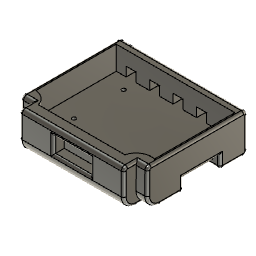
Carcasa Muñeca v10.0 (Autodesk Fusion 360 design; units mm, degrees)
Autodesk Fusion 360 part; units mm, degrees
sketch "Sketch10" plane through (0, 0, 0) normal (0, 0, 1) x (1, 0, 0)
  line L0 (0, -50) -> (0, 50) construction
  line L1 (0, 50) -> (-57, 50)
  line L2 (-57, 50) -> (-57, 0)
  line L3 (0, -50) -> (-45, -50)
  line L4 (-45, -50) -> (-45, -30)
  arc A0 (-57, 0) -> (-45, -30) centre (-7.0663, 2.5735) ccw
  line L5 (0, -50) -> (45, -50)
  line L6 (45, -50) -> (45, -30)
  arc A1 (45, -30) -> (57, 0) centre (7.0663, 2.5735) ccw
  line L7 (57, 50) -> (57, 0)
  line L8 (0, 50) -> (57, 50)
  dimension "d19" = 100
  dimension "d20" = 57
  dimension "d21" = 50
  dimension "d22" = 45
  dimension "d23" = 20
  dimension "d24" = 50
  dimension "d25" = 30
  constraint vertical L0
  constraint midpoint L0 origin
  constraint perpendicular L0 L1
  constraint perpendicular L1 L2
  constraint perpendicular L0 L3
  constraint perpendicular L3 L4
  constraint symmetric L3.start L0 L5.start
  constraint symmetric L1.start L0 L8.start
  constraint symmetric L0 L1.end L7.start
  constraint symmetric L0 L2.end A1.end
  constraint symmetric L0 L3.end L5.end
  constraint symmetric L0 L4.end L6.end
  constraint symmetric L0 A0 A1
  measures "d19" distance of L0.start L0.end
  measures "d20" distance of L0.end L1.end
  measures "d21" distance of L1.end L2.end
  measures "d22" distance of L0.start L3.end
  measures "d23" distance of L3.end L4.end
  measures "d24" radius of A0
  measures "d25" vertical distance of L2.end L4.end
sketch "Sketch12" plane through (0, 0, 0) normal (1, 0, 0) x (0, 1, 0)
  line L0 (0, 15.5) -> (0, -15.5) construction
  line L1 (0, 15.5) -> (40, 15.5)
  line L2 (43, 12.5) -> (43, -12.5)
  arc A0 (43, 12.5) -> (40, 15.5) centre (40, 12.5) ccw
  line L3 (0, 15.5) -> (-45, 15.5)
  line L4 (-48, 12.5) -> (-48, -5.5)
  arc A1 (-45, 15.5) -> (-48, 12.5) centre (-45, 12.5) ccw
  arc A2 (-48, -5.5) -> (-38, -15.5) centre (-38, -5.5) ccw
  arc A3 (40, -15.5) -> (43, -12.5) centre (40, -12.5) ccw
  line L5 (-38, -15.5) -> (40, -15.5)
  dimension "d30" = 3
  dimension "d34" = 3
  dimension "d35" = 10
  dimension "d36" = 18
  dimension "d38" = 3
  dimension "d40" = 25
  dimension "d308" = 45
  dimension "d309" = 40
  constraint vertical L0
  constraint midpoint L0 origin
  constraint perpendicular L0 L1
  constraint perpendicular L1 L2
  constraint tangent L1 A0
  constraint tangent L2 A0
  constraint perpendicular L0 L3
  constraint perpendicular L3 L4
  constraint tangent L4 A1
  constraint tangent L3 A1
  constraint tangent L4 A2
  constraint tangent L2 A3
  constraint tangent A3 L5
  measures "d30" radius of A0
  measures "d34" radius of A1
  measures "d35" radius of A2
  measures "d36" distance of L4.start L4.end
  measures "d38" radius of A3
  measures "d40" distance of L2.start L2.end
  measures "d308" distance of L0.start L3.end
  measures "d309" distance of L0.start L1.end
extrude "Extrude1" add sketch "Sketch12" along normal mid plane 84
ref_plane "PlanoDeObra18" through (-51, -2.5, 0) normal (-1, 0, 0) x (0, -1, 0)
sketch "Boceto31" plane through (-42, 0, 0) normal (-1, 0, 0) x (0, -1, 0)
  line L0 (45, 15.5) -> (-40, 15.5)
  line L1 (-43, 12.5) -> (-43, -12.5)
  arc A0 (-43, -12.5) -> (-40, -15.5) centre (-40, -12.5) ccw
  arc A1 (38, -15.5) -> (48, -5.5) centre (38, -5.5) ccw
  line L2 (48, -5.5) -> (48, 12.5)
  arc A2 (48, 12.5) -> (45, 15.5) centre (45, 12.5) ccw
  arc A3 (-43, -12.5) -> (-40, -15.5) centre (-40, -12.5) ccw
  line L3 (-40, -12.5) -> (-43, -12.5) construction
  line L4 (-40, -12.5) -> (-40, -15.5) construction
  line L5 (-40, -15.5) -> (28, -15.5)
  line L6 (-40, 15.5) -> (35, 15.5)
  line L7 (-43, 12.5) -> (-43, -12.5)
  arc A4 (38, 12.5) -> (34.9876, 15.5) centre (35, 12.5) ccw
  line L8 (35, 12.5) -> (38, 12.5) construction
  line L9 (35, 12.5) -> (34.9876, 15.5) construction
  arc A5 (28, -15.5) -> (38, -5.5) centre (28, -5.5) ccw
  line L10 (28, -5.5) -> (28, -15.5) construction
  line L11 (28, -5.5) -> (38, -5.5) construction
  line L12 (38, -5.5) -> (38, 12.5)
  line L13 (-40, -15.5) -> (38, -15.5)
  arc A6 (-40, 15.5) -> (-43, 12.4998) centre (-40, 12.5) ccw
  line L14 (-40, 12.5) -> (-40, 15.5) construction
  line L15 (-40, 12.5) -> (-43, 12.4998) construction
  dimension "d172" = 3
  dimension "d176" = 3
  dimension "d178" = 10
  dimension "d313" = 68
  dimension "d315" = 75
  dimension "d316" = 3
  dimension "d396" = 10
  constraint coincident A0.centre A3.centre
  constraint coincident A0.end A3.end
  constraint perpendicular L4 L5
  constraint parallel L0 L6
  constraint tangent A3 L7
  constraint tangent L6 A4
  constraint tangent L5 A5
  constraint tangent A5 L12
  constraint tangent A4 L12
  constraint perpendicular L6 L12
  constraint coincident L0.end L6.start
  constraint tangent L6 A6
  constraint tangent L7 A6
  measures "d172" radius of A3
  measures "d176" radius of A4
  measures "d178" radius of A5
  measures "d313" distance of A0.end L5.end
  measures "d315" distance of L0.end L6.end
  measures "d316" radius of A6
  measures "d396" distance of L2 L12
extrude "Extruir14" add sketch "Boceto31" along normal blind 9 contours L0 L1 A0 A3 L5 L6 L7 A4 A5 L12 L13 A6
sketch "Boceto32" plane through (42, 0, 0) normal (1, 0, 0) x (0, 1, 0)
  line L0 (40, 15.5) -> (-45, 15.5)
  arc A0 (-45, 15.5) -> (-48, 12.5) centre (-45, 12.5) ccw
  line L1 (-48, 12.5) -> (-48, -5.5)
  arc A1 (-48, -5.5) -> (-38, -15.5) centre (-38, -5.5) ccw
  arc A2 (40, -15.5) -> (43, -12.5) centre (40, -12.5) ccw
  line L2 (43, -12.5) -> (43, 12.5)
  arc A3 (43, 12.5) -> (40, 15.5) centre (40, 12.5) ccw
  arc A4 (43, 12.5) -> (40, 15.5) centre (40, 12.5) ccw
  line L3 (40, 12.5) -> (43, 12.5) construction
  line L4 (40, 12.5) -> (40, 15.5) construction
  line L5 (40, 15.5) -> (-35, 15.5)
  arc A5 (40, -15.5) -> (43, -12.5) centre (40, -12.5) ccw
  line L6 (40, -12.5) -> (40, -15.5) construction
  line L7 (40, -12.5) -> (43, -12.5) construction
  line L8 (-28, -15.5) -> (-28, -5.5) construction
  arc A6 (-37.9995, -5.4037) -> (-28, -15.5) centre (-28, -5.5) ccw
  line L9 (-28, -5.5) -> (-37.9995, -5.4037) construction
  line L10 (-28, -5.5) -> (-28, -15.5) construction
  arc A7 (-34.8271, 15.5) -> (-37.8271, 12.5004) centre (-34.8271, 12.5) ccw
  line L11 (-34.8271, 12.5) -> (-34.8271, 15.5) construction
  line L12 (-34.8271, 12.5) -> (-37.8271, 12.5004) construction
  line L13 (-37.8271, 12.5004) -> (-37.9995, -5.4037)
  line L14 (-28, -15.5) -> (40, -15.5)
  line L15 (-28, -15.5) -> (40, -15.5)
  line L16 (43, 12.5) -> (43, -12.5)
  dimension "d182" = 3
  dimension "d185" = 3
  dimension "d320" = 10
  dimension "d322" = 3
  dimension "d397" = 75
  dimension "d398" = 68
  constraint coincident A3.centre A4.centre
  constraint coincident L0.start A3.end
  constraint coincident A2.centre A5.centre
  constraint coincident A2.start A5.start
  constraint coincident L8.start A6.end
  constraint coincident L8.end A6.centre
  constraint tangent A6 L13
  constraint tangent L5 A7
  constraint tangent A6 L14
  measures "d182" radius of A4
  measures "d185" radius of A5
  measures "d320" radius of A6
  measures "d322" radius of A7
  measures "d397" distance of L0.start L5.end
  measures "d398" distance of A2.start L8.start
extrude "Extruir15" add sketch "Boceto32" along normal blind 9
ref_plane "PlanoDeObra19" through (0, -2.5, -0.5) normal (0, 0, 1) x (0, -1, 0)
sketch "Boceto33" plane through (0, 0, -0.5) normal (0, 0, 1) x (1, 0, 0)
  line L0 (48, 36) -> (-48, 36)
  line L1 (-48, 36) -> (-48, -29)
  line L2 (48, -29) -> (48, 36)
  line L3 (-37, -37.9882) -> (33, -37.9882)
  line L4 (-51, 40) -> (-51, -28)
  line L5 (-42, 40) -> (51, 40)
  line L6 (-42, -45) -> (42, -45)
  line L7 (-42, -45) -> (-42, -35)
  line L8 (51, 40) -> (51, -34.8271)
  arc A0 (-37, -37.9882) -> (-48, -29) centre (-48.8903, -41.3147) ccw
  arc A1 (48, -29) -> (33, -37.9882) centre (44.9809, -40.972) ccw
  line L9 (42, -34.8271) -> (42, -45)
  dimension "d257" = 3
  dimension "d310" = 4
  dimension "d325" = 70
  dimension "d327" = 65
  dimension "d330" = 3
  dimension "d399" = 5
  dimension "d400" = 9
  constraint horizontal L0
  constraint vertical L1
  constraint vertical L2
  constraint horizontal L3
  constraint equal L1 L2
  constraint equal A0 A1
  measures "d257" distance of L1 L4
  measures "d310" distance of L0 L5
  measures "d325" distance of L3.start L3.end
  measures "d327" distance of L0.end L1.end
  measures "d330" distance of L2 L8
  measures "d399" distance of L3.start L7
  measures "d400" distance of L3.end L9
extrude "Extruir16" cut sketch "Boceto33" along normal blind 16 and the other way blind 3
ref_plane "PlanoDeObra20" through (51, 2.5864, 15.5) normal (-1, 0, 0) x (0, -1, 0)
sketch "Boceto34" plane through (51, 10, 10) normal (-1, 0, 0) x (0, 0, -1)
  line L0 (25.5, 19) -> (15.5, 19)
  line L1 (15.5, 19) -> (15.5, -11)
  line L2 (15.5, -11) -> (25.5, -11)
  line L3 (25.5, -11) -> (25.5, 19)
  line L4 (25.5, 38) -> (25.5, -30)
  dimension "d205" = 10
  dimension "d206" = 30
  dimension "d331" = 19
  constraint horizontal L0
  constraint vertical L1
  constraint horizontal L2
  constraint vertical L3
  constraint coincident L2.end L4
  measures "d205" distance of L0.start L0.end
  measures "d206" distance of L0.start L2.end
  measures "d331" distance of L2 L4.end
extrude "Extruir17" cut sketch "Boceto34" along normal blind 15
ref_plane "PlanoDeObra21" through (43.5, -9, -10.5) normal (0, 1, 0) x (0, 0, -1)
sketch "Boceto35" plane through (46.5, -9, -6.0333) normal (0, 1, 0) x (1, 0, 0)
  circle A0 centre (-3, 4.4667) radius 1.5
  line L0 (4.5, -0.5333) -> (-10.5, -0.5333)
  line L1 (-10.5, 9.4667) -> (-10.5, -0.5333)
  line L2 (-10.5, 9.4667) -> (4.5, 9.4667)
  line L3 (4.5, 9.4667) -> (4.5, -0.5333)
  dimension "d210" = 3
  dimension "d290" = 5
  dimension "d291" = 7.5
  dimension "d332" = 5
  dimension "d333" = 7.5
  measures "d210" diameter of A0
  measures "d290" distance of A0.centre L0
  measures "d291" distance of A0.centre L1
  measures "d332" distance of A0.centre L2
  measures "d333" distance of A0.centre L3
extrude "Extruir18" add sketch "Boceto35" along normal up to surface (30 mm away) contours A0
sketch "Boceto43" plane through (-51, 0, 0) normal (-1, 0, 0) x (0, -1, 0)
  line L0 (38, -5.5) -> (38, 12.5)
  arc A0 (38, 12.5) -> (35, 15.5) centre (35, 12.5) ccw
  line L1 (35, 15.5) -> (-40, 15.5)
  arc A1 (-40, 15.5) -> (-43, 12.4998) centre (-40, 12.5) ccw
  line L2 (-43, 12.4998) -> (-43, -12.5)
  arc A2 (-43, -12.5) -> (-40, -15.5) centre (-40, -12.5) ccw
  line L3 (-40, -15.5) -> (28, -15.5)
  arc A3 (28, -15.5) -> (38, -5.5) centre (28, -5.5) ccw
  line L4 (-21, -15.5) -> (9, -15.5)
  line L5 (9, -15.5) -> (9, -5.5)
  line L6 (9, -5.5) -> (-21, -5.5)
  line L7 (-21, -5.5) -> (-21, -15.5)
  dimension "d360" = 30
  dimension "d361" = 10
  dimension "d401" = 19
  constraint horizontal L4
  constraint vertical L5
  constraint horizontal L6
  constraint vertical L7
  constraint coincident L3 L4.start
  measures "d360" distance of L4.start L4.end
  measures "d361" distance of L4.start L6.end
  measures "d401" distance of A2.end L4.start
extrude "Extruir26" cut sketch "Boceto43" against normal blind 15 contours L3 L4 L5 L6 L7
sketch "Boceto44" plane through (0, -9, 0) normal (0, 1, 0) x (-1, 0, 0)
  line L0 (51, -15.5) -> (51, -5.5)
  line L1 (51, -5.5) -> (36, -5.5)
  line L2 (36, -5.5) -> (36, -15.5)
  line L3 (36, -15.5) -> (51, -15.5)
  circle A0 centre (43.5, -10.5) radius 1.5
  dimension "d365" = 3
  dimension "d366" = 7.5
  dimension "d367" = 7.5
  dimension "d368" = 5
  dimension "d369" = 5
  measures "d365" diameter of A0
  measures "d366" distance of L2 A0.centre
  measures "d367" distance of L0 A0.centre
  measures "d368" distance of L1 A0.centre
  measures "d369" distance of L3 A0.centre
extrude "Extruir27" add sketch "Boceto44" along normal up to surface (30 mm away) contours A0
ref_plane "PlanoDeObra22" through (-51, 2.5, 0) normal (-1, 0, 0) x (0, -1, 0)
ref_plane "PlanoDeObra23" through (0, 43, 0) normal (0, 1, 0) x (0, 0, 1)
ref_plane "PlanoDeObra25" through (0, -48, 3.5) normal (0, -1, 0) x (0, 0, -1)
sketch "Boceto36" plane through (0, -48, 3.5) normal (0, -1, 0) x (1, 0, 0)
  line L0 (-14.9998, 6) -> (15.0002, 6)
  line L1 (15.0002, 6) -> (15.0002, -7)
  line L2 (15.0002, -7) -> (-14.9998, -7)
  line L3 (-14.9998, -7) -> (-14.9998, 6)
  line L4 (-14.9998, 6) -> (15.0002, -7) construction
  line L5 (15.0002, 6) -> (-14.9998, -7) construction
  line L6 (-42, -9) -> (42, -9)
  line L7 (-42, 9) -> (42, 9)
  point P0 (0.0002, -0.5)
  dimension "d217" = 30
  dimension "d218" = 13
  dimension "d335" = 3
  constraint horizontal L0
  constraint perpendicular L0 L1
  constraint parallel L0 L2
  constraint parallel L1 L3
  constraint coincident L4 P0
  constraint coincident L5 P0
  measures "d217" distance of L1.end L2.end
  measures "d218" distance of L0.end L1.end
  measures "d335" distance of L0 L7
extrude "Extruir19" cut sketch "Boceto36" against normal blind 9
fillet "Empalme13" radius 2 9 edges at (-51, 43, -0.0001) (-51, 42.1213, -14.6213) (-51, -18.5, -15.5) (-51, 30.5, -15.5) (-51, -35.0711, -12.5711) (-51, -38, 3.5) (-51, -37.1213, 14.6213) (-51, 2.5, 15.5) (-51, 42.1214, 14.6212)
fillet "Empalme14" radius 2 5 edges at (-42, -33, -15.5) (-42, -45.0711, -12.5711) (-42, -48, 3.5) (-42, -47.1213, 14.6213) (-42, -40, 15.5)
fillet "Empalme15" radius 2 9 edges at (51, 30.5, -15.5) (51, 42.1213, -14.6213) (51, 43, 0) (51, 42.1213, 14.6213) (51, 2.5864, 15.5) (51, -36.9483, 14.6215) (51, -37.9133, 3.5484) (51, -35.105, -12.5369) (51, -18.5, -15.5)
fillet "Empalme16" radius 2 5 edges at (42, -39.9136, 15.5) (42, -47.1213, 14.6213) (42, -48, 3.5) (42, -45.0711, -12.5711) (42, -33, -15.5)
sketch "Boceto39" plane through (0, 43, 0) normal (0, 1, 0) x (1, 0, 0)
  line L0 (44, 3.5) -> (36, 3.5)
  line L1 (36, 3.5) -> (36, -4)
  line L2 (36, -4) -> (44, -4)
  line L3 (44, -4) -> (44, 3.5)
  line L4 (49, 12.5771) -> (49, -12.4229)
  line L5 (25, 3.5) -> (17, 3.5)
  line L6 (17, 3.5) -> (17, -4)
  line L7 (17, -4) -> (25, -4)
  line L8 (25, -4) -> (25, 3.5)
  line L9 (6, 3.5) -> (-2, 3.5)
  line L10 (-2, 3.5) -> (-2, -4)
  line L11 (-2, -4) -> (6, -4)
  line L12 (6, -4) -> (6, 3.5)
  line L13 (-13, 3.5) -> (-21, 3.5)
  line L14 (-21, 3.5) -> (-21, -4)
  line L15 (-21, -4) -> (-13, -4)
  line L16 (-13, -4) -> (-13, 3.5)
  line L17 (-32, 3.5) -> (-40, 3.5)
  line L18 (-40, 3.5) -> (-40, -4)
  line L19 (-40, -4) -> (-32, -4)
  line L20 (-32, -4) -> (-32, 3.5)
  line L21 (-42, -12.5) -> (49, -12.5)
  line L22 (-49, -12.4998) -> (-49, 12.5)
  line L23 (49, 3.6424) -> (-49, 3.6424)
  line L24 (49, 12.5) -> (49, -12.5)
  dimension "d236" = 8
  dimension "d237" = 7.5
  dimension "d239" = 8
  dimension "d240" = 7.5
  dimension "d242" = 8
  dimension "d243" = 7.5
  dimension "d245" = 8
  dimension "d246" = 7.5
  dimension "d248" = 8
  dimension "d249" = 7.5
  dimension "d280" = 11
  dimension "d281" = 11
  dimension "d282" = 11
  dimension "d285" = 11
  dimension "d373" = 5
  dimension "d374" = -9
  constraint horizontal L0
  constraint vertical L1
  constraint horizontal L2
  constraint vertical L3
  constraint horizontal L5
  constraint vertical L6
  constraint horizontal L7
  constraint vertical L8
  constraint horizontal L9
  constraint vertical L10
  constraint horizontal L11
  constraint vertical L12
  constraint horizontal L13
  constraint vertical L14
  constraint horizontal L15
  constraint vertical L16
  constraint horizontal L17
  constraint vertical L18
  constraint horizontal L19
  constraint vertical L20
  constraint coincident L4 L23.start
  constraint coincident L22 L23.end
  constraint perpendicular L22 L23
  constraint coincident L23.start L24
  measures "d236" distance of L0.start L0.end
  measures "d237" distance of L0.start L2.end
  measures "d239" distance of L5.start L5.end
  measures "d240" distance of L5.start L7.end
  measures "d242" distance of L9.start L9.end
  measures "d243" distance of L9.start L11.end
  measures "d245" distance of L13.start L13.end
  measures "d246" distance of L13.start L15.end
  measures "d248" distance of L17.start L17.end
  measures "d249" distance of L17.start L19.end
  measures "d280" distance of L1 L8
  measures "d281" distance of L6 L12
  measures "d282" distance of L10 L16
  measures "d285" distance of L14 L20
  measures "d373" distance of L3 L4
  measures "d374" distance of L17.end L22
extrude "Extruir22" cut sketch "Boceto39" against normal blind 8
sketch "Boceto40" plane through (0, 0, -3.5) normal (0, 0, 1) x (-1, 0, 0)
  line L0 (48, -36) -> (48, 29)
  line L1 (37, 37.9882) -> (-33, 37.9882)
  line L2 (-48, 29) -> (-48, -36)
  line L3 (-48, -36) -> (-44, -36)
  line L4 (-44, -36) -> (-44, -43)
  line L5 (-44, -43) -> (-36, -43)
  line L6 (-36, -43) -> (-36, -36)
  line L7 (-36, -36) -> (-25, -36)
  line L8 (-25, -36) -> (-25, -43)
  line L9 (-25, -43) -> (-17, -43)
  line L10 (-17, -43) -> (-17, -36)
  line L11 (-17, -36) -> (-6, -36)
  line L12 (-6, -36) -> (-6, -43)
  line L13 (-6, -43) -> (2, -43)
  line L14 (2, -43) -> (2, -36)
  line L15 (2, -36) -> (13, -36)
  line L16 (13, -36) -> (13, -43)
  line L17 (13, -43) -> (21, -43)
  line L18 (21, -43) -> (21, -36)
  line L19 (21, -36) -> (32, -36)
  line L20 (32, -36) -> (32, -43)
  line L21 (32, -43) -> (40, -43)
  line L22 (40, -43) -> (40, -36)
  line L23 (40, -36) -> (48, -36)
  arc A0 (-48, 29) -> (-33, 37.9882) centre (-44.9809, 40.972) ccw
  arc A1 (37, 37.9882) -> (48, 29) centre (48.8903, 41.3147) ccw
sketch "Boceto41" plane through (0, 0, -3.5) normal (0, 0, 1) x (1, 0, 0)
  circle A0 centre (-31.95, 26) radius 1.55
  circle A1 centre (-31.95, -14.2) radius 1.55
  circle A2 centre (31.95, 26) radius 1.55
  circle A3 centre (31.95, -14.2) radius 1.55
  line L0 (31.95, -14.2) -> (-31.95, -14.2)
  line L1 (-31.95, -14.2) -> (-31.95, 26)
  line L2 (-31.95, 26) -> (31.95, 26)
  line L3 (31.95, 26) -> (31.95, -14.2)
  line L4 (-48, -29) -> (-48, 36)
  line L5 (48, 36) -> (48, -29)
  line L6 (-48, 36) -> (48, 36)
  line L7 (33, -37.9882) -> (-37, -37.9882)
  dimension "d260" = 3.1
  dimension "d261" = 3.1
  dimension "d262" = 3.1
  dimension "d266" = 3.1
  dimension "d267" = 63.9
  dimension "d268" = 40.2
  dimension "d375" = 16.05
  dimension "d377" = 10
  dimension "d395" = 16.05
  dimension "d402" = 23.7882
  constraint coincident A3.centre L0.start
  constraint coincident A1.centre L0.end
  constraint horizontal L0
  constraint coincident A0.centre L1.end
  constraint perpendicular L0 L1
  constraint coincident A2.centre L2.end
  measures "d260" diameter of A0
  measures "d261" diameter of A1
  measures "d262" diameter of A2
  measures "d266" diameter of A3
  measures "d267" distance of A1.centre A3.centre
  measures "d268" distance of A2.centre A3.centre
  measures "d375" distance of A0.centre L4
  measures "d377" distance of L2 L6
  measures "d395" distance of L3 L5
  measures "d402" distance of L0 L7
extrude "Extruir23" cut sketch "Boceto41" against normal blind 12 contours A0 L1 L2 | A0 L1 L2 | A2 L2 L3 | A2 L2 L3 | A1 L0 L1 | A1 L0 L1 | A3 L0 L3 | A3 L0 L3
fillet "Empalme19" radius 2 8 edges at (36, 6, -15.5) (42.5, -9, -15.5) (50.4142, -9, -14.9142) (51, -9, -9.5) (51, 21, -9.5) (50.4142, 21, -14.9142) (42.5, 21, -15.5) (51, 6, -5.5)
fillet "Empalme20" radius 2 8 edges at (-51, 6, -5.5) (-51, -9, -9.5) (-50.4142, -9, -14.9142) (-42.5, -9, -15.5) (-42.5, 21, -15.5) (-50.4142, 21, -14.9142) (-51, 21, -9.5) (-36, 6, -15.5)
fillet "Empalme21" radius 2 4 edges at (0.0002, -48, -3.5) (-14.9998, -48, 3) (0.0002, -48, 9.5) (15.0002, -48, 3)
sketch "Boceto45" plane through (0, 0, -15.5) normal (0, 0, -1) x (1, 0, 0)
  line L0 (-34, -23) -> (-49, -23)
  line L1 (-49, -23) -> (-49, -40)
  line L2 (-49, -40) -> (49, -40)
  line L3 (49, -40) -> (49, -23)
  line L4 (49, -23) -> (34, -23)
  line L5 (34, -23) -> (34, 11)
  line L6 (34, 11) -> (49, 11)
  line L7 (49, 11) -> (49, 28)
  line L8 (49, 28) -> (40, 28)
  line L9 (40, 28) -> (40, 38)
  line L10 (40, 38) -> (-40, 38)
  line L11 (-40, 38) -> (-40, 28)
  line L12 (-40, 28) -> (-49, 28)
  line L13 (-49, 28) -> (-49, 11)
  line L14 (-49, 11) -> (-34, 11)
  line L15 (-34, 11) -> (-34, -23)
  circle A0 centre (-31.95, 14.2) radius 1.55
  circle A1 centre (31.95, -26) radius 1.55
  circle A2 centre (-31.95, -26) radius 1.55
  circle A3 centre (31.95, 14.2) radius 1.55
  circle A4 centre (31.95, -26) radius 3.5
  circle A5 centre (31.95, 14.2) radius 3.5
  circle A6 centre (-31.95, -26) radius 3.5
  circle A7 centre (-31.95, 14.2) radius 3.5
  dimension "d385" = 7
  dimension "d386" = 7
  dimension "d387" = 7
  dimension "d388" = 7
  constraint concentric A1 A4
  constraint concentric A3 A5
  constraint concentric A2 A6
  constraint concentric A0 A7
  measures "d385" diameter of A4
  measures "d386" diameter of A5
  measures "d387" diameter of A6
  measures "d388" diameter of A7
extrude "Extruir29" cut sketch "Boceto45" against normal blind 2.5 contours A4 | A5 | A6 | A7
fillet "Empalme23" radius 1 4 edges at (28.6869, 24.7343, -15.5) (28.6869, -15.4657, -15.5) (-35.2131, -15.4657, -15.5) (-35.2131, 24.7343, -15.5)
